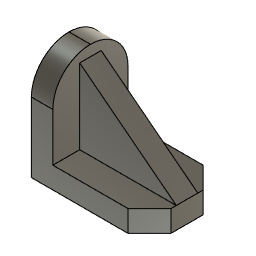
A1 v1 (Autodesk Fusion 360 design; units mm, degrees)
Autodesk Fusion 360 part; units mm, degrees
sketch "base" plane through (0, 0, 0) normal (0, 0, 1) x (1, 0, 0)
  line L0 (-19.5692, -20.5967) -> (46.4308, -20.5967)
  line L1 (46.4308, -20.5967) -> (46.4308, 21.4033)
  line L2 (46.4308, 21.4033) -> (-19.5692, 21.4033)
  line L3 (-19.5692, 21.4033) -> (-19.5692, -20.5967)
  line L4 (46.4308, -20.5967) -> (46.4308, -8.5967)
  line L5 (46.4308, -20.5967) -> (34.4308, -20.5967)
  line L6 (46.4308, -8.5967) -> (34.4308, -20.5967)
  line L7 (46.4308, 9.4033) -> (34.4308, 21.4033)
  line L8 (46.4308, 21.4033) -> (34.4308, 21.4033)
  line L9 (46.4308, 21.4033) -> (46.4308, 9.4033)
  line L10 (-19.5692, 21.4033) -> (-7.5692, 21.4033)
  line L11 (-19.5692, -20.5967) -> (-7.5692, -20.5967)
  line L12 (-7.5692, 21.4033) -> (-7.5692, -20.5967)
  dimension "d1" = 66
  dimension "d2" = 42
  dimension "d3" = 12
  dimension "d4" = 12
  constraint horizontal L0
  constraint vertical L1
  constraint horizontal L2
  constraint vertical L3
  constraint perpendicular L0 L4
  constraint perpendicular L1 L5
  constraint perpendicular L11 L12
  measures "d1" distance of L0.start L0.end
  measures "d2" distance of L0.start L2.end
  measures "d3" distance of L0.end L4.end
  measures "d4" distance of L0.end L5.end
extrude "Extrude1" add sketch "base" along normal blind 12 contours L0 L1 L2 L6 L7 L12
extrude "Extrude2" add sketch "base" along normal blind 39 contours L0 L2 L3 L10 L11 L12
sketch "ramp" plane through (0, 0, 12) normal (0, 0, 1) x (-1, 0, 0)
  line L0 (-46.4308, 8.5967) -> (-46.4308, -9.4033)
  line L1 (-46.4308, -9.4033) -> (-34.4308, -21.4033)
  line L2 (-34.4308, -21.4033) -> (7.5692, -21.4033)
  line L3 (7.5692, -21.4033) -> (7.5692, 20.5967)
  line L4 (7.5692, 20.5967) -> (-34.4308, 20.5967)
  line L5 (-34.4308, 20.5967) -> (-46.4308, 8.5967)
  line L6 (7.5692, -21.4033) -> (7.5692, -6.4033)
  line L7 (7.5692, 20.5967) -> (7.5692, 5.5967)
  line L8 (7.5692, -6.4033) -> (-46.4308, -6.4033)
  line L9 (7.5692, 5.5967) -> (-46.4308, 5.5967)
  dimension "d9" = 15
  dimension "d10" = 15
  constraint coincident L2.end L3.start
  constraint perpendicular L2 L6
  constraint coincident L3.end L4.start
  constraint perpendicular L4 L7
  constraint coincident L0 L8.end
  constraint perpendicular L0 L8
  constraint coincident L0 L9.end
  constraint perpendicular L0 L9
  measures "d9" distance of L2.end L6.end
  measures "d10" distance of L3.end L7.end
extrude "Extrude3" add sketch "ramp" along normal blind 42 contours L0 L3 L8 L9
sketch "triangle" plane through (0, -5.5967, 0) normal (0, -1, 0) x (1, 0, 0)
  line L0 (-7.5692, 12) -> (46.4308, 12)
  line L1 (46.4308, 12) -> (46.4308, 54)
  line L2 (46.4308, 54) -> (-7.5692, 54)
  line L3 (-7.5692, 54) -> (-7.5692, 39)
  line L4 (-7.5692, 39) -> (-7.5692, 12)
  line L5 (-7.5692, 54) -> (46.4308, 12)
  line L6 (-7.5692, 54) -> (46.4308, 54)
  line L7 (46.4308, 12) -> (46.4308, 54)
  constraint coincident L2.end L3.start
  constraint coincident L0.end L1.start
  constraint coincident L1.end L2.start
extrude "Extrude4" cut sketch "triangle" against normal blind 12 contours L1 L2 L5 L6 L7
extrude "Extrude5" add 1 faces at (-15.5692, -1.5967, 39) along direction (0, 0, 1) blind 21
sketch "round" plane through (-7.5692, 0, 0) normal (1, 0, 0) x (0, 1, 0)
  line L0 (6.4033, 54) -> (6.4033, 12)
  line L1 (6.4033, 12) -> (21.4033, 12)
  line L2 (21.4033, 12) -> (21.4033, 60)
  line L3 (21.4033, 60) -> (-20.5967, 60)
  line L4 (-20.5967, 60) -> (-20.5967, 12)
  line L5 (-20.5967, 12) -> (-5.5967, 12)
  line L6 (-5.5967, 12) -> (-5.5967, 54)
  line L7 (-5.5967, 54) -> (6.4033, 54)
  line L8 (-20.5967, 12) -> (-20.5967, 39)
  arc A0 (0.4033, 60) -> (-20.5967, 39) centre (0.4033, 39) ccw
  line L9 (21.4033, 12) -> (21.4033, 39)
  arc A1 (21.4033, 39) -> (0.4033, 60) centre (0.4033, 39) ccw
  line L10 (21.4033, 39) -> (21.4033, 60)
  line L11 (0.4033, 60) -> (-20.5967, 60)
  line L12 (-20.5967, 39) -> (-20.5967, 60)
  dimension "d17" = 27
  dimension "d18" = 27
  constraint coincident L4.end L5.start
  constraint perpendicular L5 L8
  constraint midpoint L3 A0.start
  constraint tangent L8 A0
  constraint coincident L1.end L2.start
  constraint coincident L2 L9.end
  constraint tangent L9 A1
  constraint coincident L2.end L3.start
  constraint coincident L3.end L4.start
  constraint tangent A0 L11
  measures "d17" distance of L4.end L8.end
  measures "d18" distance of L1.end L9.end
extrude "Extrude8" cut sketch "round" against normal blind 12 contours L2 L3 A1 L10
extrude "Extrude6" cut sketch "round" against normal blind 12 contours L2 L3 A1 L10
extrude "Extrude7" cut sketch "round" against normal blind 12 contours L3 L4 A0 L11 L12
